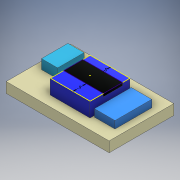
# Autodesk Inventor part: placa electronica optiweather
Saved by Autodesk Inventor 2017 (Build 210142000, 142)
## iProperties
Part Number: placa electronica optiweather
Material: Genérico
Document SubType Name: Modeling
Designer: user
Density: 1 g/cm^3
Appearance: Valor por defecto
Author: user
Autodesk Inventor part; units mm, degrees
ref_plane "YZ Plane" through (0, 0, 0) normal (1, 0, 0) x (0, 1, 0)
ref_plane "XZ Plane" through (0, 0, 0) normal (0, 1, 0) x (-1, 0, 0)
ref_plane "XY Plane" through (0, 0, 0) normal (0, 0, 1) x (1, 0, 0)
sketch "Boceto1" plane through (0, 0, 0) normal (0, 0, 1) x (1, 0, 0)
  line L0 (35, 22) -> (-35, 22)
  line L1 (-35, 22) -> (-35, -22)
  line L2 (-35, -22) -> (35, -22)
  line L3 (35, -22) -> (35, 22)
  point P0 (0, 0)
  point P1 (35, 0)
  point P2 (0, 22)
  dimension "d0" = 70
  dimension "d1" = 44
  constraints: 8 end point, 2 midpoint, 2 parallel, 1 horizontal, 1 horizontal alignment, 1 perpendicular, 1 vertical alignment
  measures "d0" distance of L1.end L2.end
  measures "d1" distance of L2.end L0.start
extrude "Extrusión1" add sketch "Boceto1" along normal blind 7
sketch "Boceto2" plane through (0, 0, 7) normal (0, 0, 1) x (1, 0, 0)
  line L0 (35, 22) -> (-35, 22) construction
  line L1 (-35, 22) -> (-35, -22) construction
  line L2 (-35, -22) -> (35, -22) construction
  line L3 (35, -22) -> (35, 22) construction
  line L4 (-35, 22) -> (-35, -22) construction
  line L5 (-35, 22) -> (-35, 15) construction
  line L6 (-35, 15) -> (-30, 15) construction
  line L7 (-30, 15) -> (-30, -3)
  line L8 (-30, -3) -> (-19, -3)
  line L9 (-19, -3) -> (-19, 15)
  line L10 (-19, 15) -> (-30, 15)
  line L11 (-35, 22) -> (-12, 22) construction
  line L12 (-12, 22) -> (-12, 12) construction
  line L13 (-12, 12) -> (-12, -15)
  line L14 (-12, -15) -> (15, -15)
  line L15 (15, -15) -> (15, 12)
  line L16 (15, 12) -> (-12, 12)
  line L17 (35, 22) -> (-35, 22) projected
  line L18 (35, 22) -> (35, 12) construction
  line L19 (35, -22) -> (35, 22) construction
  line L20 (35, 12) -> (30, 12) construction
  line L21 (30, 12) -> (16, 12)
  line L22 (16, 12) -> (16, -13)
  line L23 (16, -13) -> (30, -13)
  line L24 (30, -13) -> (30, 12)
  point P0 (0, 0)
  dimension "d4" = 7
  dimension "d5" = 5
  dimension "d6" = 18
  dimension "d7" = 11
  dimension "d8" = 23
  dimension "d9" = 10
  dimension "d10" = 27
  dimension "d11" = 27
  dimension "d12" = 10
  dimension "d13" = 5
  dimension "d14" = 14
  dimension "d15" = 25
  dimension "d16" = 14
  constraints: 36 end point, 6 perpendicular, 4 horizontal, 4 vertical, 3 point on line
  measures "d4" distance of L0.end L5.end
  measures "d5" distance of L5.end L6.end
  measures "d6" distance of L6.end L7.end
  measures "d7" distance of L7.end L8.end
  measures "d8" distance of L0.end L11.end
  measures "d9" distance of L11.end L12.end
  measures "d10" distance of L12.end L13.end
  measures "d11" distance of L13.end L14.end
  measures "d12" distance of L0.start L18.end
  measures "d13" distance of L18.end L20.end
  measures "d14" distance of L20.end L21.end
  measures "d15" distance of L21.end L22.end
  measures "d16" distance of L22.end L23.end
extrude "Extrusión2" add sketch "Boceto2" along normal blind 5 contours L24 L23 L22 L21
extrude "Extrusión3" add sketch "Boceto2" along normal blind 10 contours L16 L15 L14 L13
extrude "Extrusión4" add sketch "Boceto2" along normal blind 6.5 contours L10 L9 L8 L7
sketch "Boceto3" plane through (0, 0, 17) normal (0, 0, 1) x (1, 0, 0)
  point P0 (0, 0)
sketch "Boceto4" plane through (0, 0, 17) normal (0, 0, 1) x (1, 0, 0)
  line L0 (-12, 12) -> (-12, -15) projected
  line L1 (-12, -15) -> (15, -15) projected
  line L2 (15, -15) -> (15, 12) projected
  line L3 (15, 12) -> (-12, 12) projected
  line L4 (-12, 12) -> (-12, -15) projected
  line L5 (15, -15) -> (15, 12) projected
  line L6 (-12, 7) -> (15, 7)
  line L7 (15, 7) -> (15, -6)
  line L8 (15, -6) -> (-12, -6)
  line L9 (-12, -6) -> (-12, 7)
  point P0 (0, 0)
  dimension "d23" = 5
  dimension "d24" = 9
  constraints: 8 end point, 2 parallel, 2 point on line, 1 horizontal, 1 perpendicular
  measures "d23" distance between parallel lines of L6 L3
  measures "d24" distance between parallel lines of L8 L1
extrude "Extrusión5" cut sketch "Boceto4" against normal blind 2 contours L6 L2 L8 L0
extrude "Extrusión6" add sketch "Boceto4" against normal blind 2 separate body contours L6 L2 L8 L0
